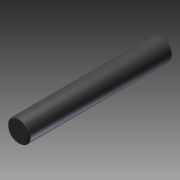
# Autodesk Inventor part: HHPSJC5-pin
Saved by Autodesk Inventor 2011 SP1 (Build 150282100, 282)
## iProperties
Created: 2015-01-26
Part Number: HHPSJC5-pin
Catalog Web Link: www.cadenas.de
Description: HHPSJC-pin-Aluminum Detachable Hinges
Vendor: MISUMI
Document SubType Name: Modeling
Designer: PARTuser1
Manufacturer: MISUMI
Mass: 0.627707 g
Surface Area: 5.3814 cm^2
Volume: 0.627707 cm^3
Density: 1 g/cm^3
Category: PARTsolutions
Company: MISUMI
Title: HHPSJC5-pin
Author: Cadenas PARTsolutions
Comments: Aluminum Detachable Hinges
PSOL_IDENT_0: {\\10.0.0.236\data_v8\23d-libs\misumi\metric\39_accessories_for_al_extrusions\hhpsjc_pin.prj},168 {V
PSOL_IDENT_1: TYP=3D},{NB=HHPSJC5-pin},{LINA=HHPSJC5-pin},{NN=HHPSJC-pin},{DATE=17.11.2014 05:31:05},{GEOMDATE=26.
PSOL_IDENT_2: 11.2008 06:11:00},{VERSION=},{LINEID=10},{LINESUBID=-1},{WBVAR=}  {NB=HHPSJC5-pin},{LINA=HHPSJC5-pin
PSOL_IDENT_3: },{KT=DUMMY},{PN=HHPSJC5},{TYPE=HHPSJC},{MATS=304 Stainless Steel},{NO=5},{L=32},{R=5.0}
SUPPLIER: MISUMI
ARTICLENO: HHPSJC5-pin
BOMINFO: HHPSJC5-pin
CREATOR: CADENAS GmbH
Autodesk Inventor part; units mm, degrees
ref_plane "YZ Plane" through (0, 0, 0) normal (1, 0, 0) x (0, 1, 0)
ref_plane "XZ Plane" through (0, 0, 0) normal (0, 1, 0) x (-1, 0, 0)
ref_plane "XY Plane" through (0, 0, 0) normal (0, 0, 1) x (1, 0, 0)
sketch "Sketch_1" plane through (0, 0, 0) normal (0, 0, 1) x (1, 0, 0)
  line L0 (0, -16) -> (0, 16)
  line L1 (0, 16) -> (2.3, 16)
  line L2 (2.3, 16) -> (2.5, 15.8)
  line L3 (2.5, 15.8) -> (2.5, -15.8)
  line L4 (2.5, -15.8) -> (2.3, -16)
  line L5 (2.3, -16) -> (0, -16)
  line L6 (0, -16) -> (0, 16)
  constraints: 14 end point
revolve "Revolution1" add sketch "Sketch_1" angle 360 about axis through (0, -16, 0) along (0, -1, 0)
ref_plane "hhpsjc_pin_XY" through (0, 0, 0) normal (0, 1, 0) x (1, 0, 0)
ref_plane "hhpsjc_pin_YZ" through (0, 0, 0) normal (1, 0, 0) x (0, 0, -1)
ref_plane "hhpsjc_pin_ZX" through (0, 0, 0) normal (0, 0, -1) x (0, 1, 0)
body "Solid1"
